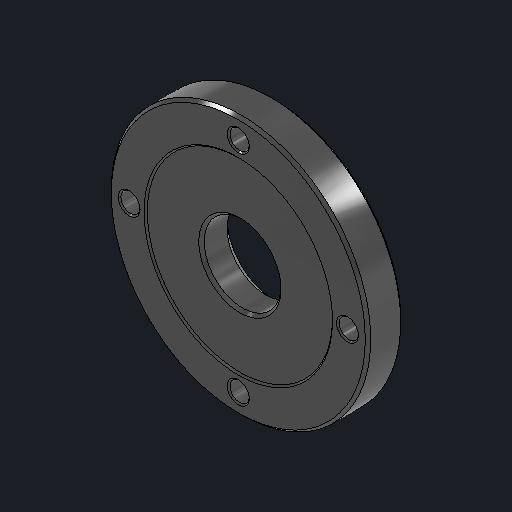
# Autodesk Inventor part: akf-60-nw25
Saved by Autodesk Inventor 2026 (Build 300175050, 175E)
## iProperties
Created: 2025-12-19
Part Number: akf-60-nw25
Material: ABS Plastic
Document SubType Name: Modeling
Designer: queezz
Density: 1.06 g/cm^3
Appearance: Dark Gray
Author: queezz
Autodesk Inventor part; units mm, degrees
ref_plane "YZ Plane" through (0, 0, 0) normal (1, 0, 0) x (0, 1, 0)
ref_plane "XZ Plane" through (0, 0, 0) normal (0, 1, 0) x (-1, 0, 0)
ref_plane "XY Plane" through (0, 0, 0) normal (0, 0, 1) x (1, 0, 0)
sketch "Sketch1" plane through (0, 0, 0) normal (0, 0, 1) x (1, 0, 0)
  circle A0 centre (0, 0) radius 28
  circle A1 centre (0, 0) radius 47.5
  dimension "d0" = 56
  dimension "d1" = 95
  constraints: 2 centre point, 2 coincident
  measures "d0" diameter of A0
  measures "d1" diameter of A1
extrude "Extrusion1" add sketch "Sketch1" along normal blind 13 contours A0 | A1
sketch "Sketch7" plane through (0, 0, 13) normal (0, 0, 1) x (1, 0, 0)
  circle A0 centre (0, 0) radius 14.05
  dimension "d42" = 28.1
  constraints: 1 centre point, 1 coincident
  measures "d42" diameter of A0
extrude "Fi28" cut sketch "Sketch7" against normal through all
sketch "Sketch2" plane through (0, 0, 0) normal (0, 0, 1) x (1, 0, 0)
  circle A0 centre (0, 0) radius 40 construction
  point P0 (40, 0)
  dimension "d4" = 80
  constraints: 2 horizontal alignment, 1 coincident, 2 other
hole "Hole1" at (40, 0, 0) direction (0, 0, 1) diameter 7 end through all counterbore diameter 11 counterbore depth 6.3
chamfer "Chamfer2" distance 0.5 angle 45 3 edges at (40, -3.5, 6.3) (40, -5.5, 0) (40, -3.5, 13)
sketch "Sketch9" plane through (40, 0, 6.3) normal (0, 0, -1) x (-1, 0, 0)
  line L0 (-4, 3.7749) -> (-4, -3.7749)
  line L1 (4, 3.7749) -> (4, -3.7749)
  line L2 (-3.7749, 4) -> (3.7749, 4)
  line L3 (3.7749, -4) -> (-3.7749, -4)
  circle A0 centre (0, 0) radius 4 projected
  circle A1 centre (0, 0) radius 5.5 projected
  point P0 (40, 0)
  constraints: 8 end point, 4 tangent, 2 parallel, 1 horizontal, 1 vertical, 9 other
extrude "Extrusion6" add sketch "Sketch9" along normal blind 0.3 contours L0 A1 | A1 L2 | L3 A1 | L1 A1
pattern_circular "Circular Pattern1" count 4 over 360 about axis through (0, 0, 0) along (0, 0, 1) of "Hole1", "Chamfer2", "Extrusion6"
chamfer "Chamfer6" distance 1 angle 45 2 edges at (-47.5, 0, 13) (-47.5, 0, 0)
sketch "Sketch10" plane through (0, 0, 13) normal (0, 0, 1) x (1, 0, 0)
  circle A0 centre (0, 0) radius 34.5
  circle A1 centre (0, 0) radius 14.05 projected
  dimension "d56" = 69
  constraints: 1 centre point, 1 coincident
  measures "d56" diameter of A0
extrude "Extrusion7" cut sketch "Sketch10" against normal blind 0.6 contours A0 | A1
chamfer "Chamfer7" distance 0.6 angle 45 1 edges at (-34.5, 0, 12.4)
chamfer "Chamfer8" distance 3 angle 45 1 edges at (-14.05, 0, 0)
chamfer "Chamfer9" distance 1 angle 45 1 edges at (-14.05, 0, 12.4)
body "Solid1"
